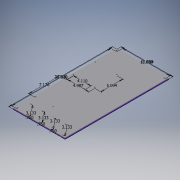
# Autodesk Inventor part: eboardbaseplate
Saved by Autodesk Inventor 2016 (Build 200138000, 138)
## iProperties
Created: 2016-01-21
Part Number: eboardbaseplate
Material: Generic
Document SubType Name: Modeling
Designer: Administrator
Density: 1 g/cm^3
Appearance: Default
Author: Administrator
Autodesk Inventor part; units mm, degrees
ref_plane "YZ Plane" through (0, 0, 0) normal (1, 0, 0) x (0, 1, 0)
ref_plane "XZ Plane" through (0, 0, 0) normal (0, 1, 0) x (-1, 0, 0)
ref_plane "XY Plane" through (0, 0, 0) normal (0, 0, 1) x (1, 0, 0)
sketch "Sketch1" plane through (0, 0, 0) normal (0, 1, 0) x (-1, 0, 0)
  line L0 (-139.7, 292.1) -> (139.7, 292.1)
  line L1 (139.7, 292.1) -> (139.7, -292.1)
  line L2 (139.7, -292.1) -> (-139.7, -292.1)
  line L3 (-139.7, -292.1) -> (-139.7, -89.789)
  line L4 (-139.7, 292.1) -> (139.7, -292.1) construction
  line L5 (139.7, 292.1) -> (-139.7, -292.1) construction
  line L6 (-152.4, 304.8) -> (152.4, 304.8)
  line L7 (152.4, 304.8) -> (152.4, -304.8)
  line L8 (152.4, -304.8) -> (-152.4, -304.8)
  line L9 (-152.4, -304.8) -> (-152.4, -89.789)
  line L10 (-152.4, 304.8) -> (152.4, -304.8) construction
  line L11 (152.4, 304.8) -> (-152.4, -304.8) construction
  line L12 (40.5945, 180.2806) -> (144.9885, 180.2806)
  line L13 (144.9885, 180.2806) -> (144.9885, -1.9898)
  line L14 (144.9885, -1.9898) -> (40.5945, -1.9898)
  line L15 (40.5945, -1.9898) -> (40.5945, 180.2806)
  line L16 (40.5945, 180.2806) -> (144.9885, -1.9898) construction
  line L17 (144.9885, 180.2806) -> (40.5945, -1.9898) construction
  line L18 (145.8849, -184.8763) -> (19.2151, -184.8763)
  line L19 (19.2151, -184.8763) -> (19.2151, -55.4887)
  line L20 (19.2151, -55.4887) -> (145.8849, -55.4887)
  line L21 (145.8849, -55.4887) -> (145.8849, -184.8763)
  line L22 (145.8849, -184.8763) -> (19.2151, -55.4887) construction
  line L23 (19.2151, -184.8763) -> (145.8849, -55.4887) construction
  line L24 (122.3815, 294.9298) -> (73.9219, 294.9298)
  line L25 (73.9219, 294.9298) -> (73.9219, 231.8081)
  line L26 (73.9219, 231.8081) -> (122.3815, 231.8081)
  line L27 (122.3815, 231.8081) -> (122.3815, 294.9298)
  line L28 (122.3815, 294.9298) -> (73.9219, 231.8081) construction
  line L29 (54.8719, 294.9298) -> (6.4122, 294.9298)
  line L30 (6.4122, 294.9298) -> (6.4122, 231.8081)
  line L31 (6.4122, 231.8081) -> (54.8719, 231.8081)
  line L32 (54.8719, 231.8081) -> (54.8719, 294.9298)
  line L33 (-12.6378, 294.9298) -> (-61.0974, 294.9298)
  line L34 (-61.0974, 294.9298) -> (-61.0974, 231.8081)
  line L35 (-61.0974, 231.8081) -> (-12.6378, 231.8081)
  line L36 (-12.6378, 231.8081) -> (-12.6378, 294.9298)
  line L37 (-80.1474, 294.9298) -> (-128.607, 294.9298)
  line L38 (-128.607, 294.9298) -> (-128.607, 231.8081)
  line L39 (-128.607, 231.8081) -> (-80.1474, 231.8081)
  line L40 (-80.1474, 231.8081) -> (-80.1474, 294.9298)
  line L41 (73.9219, 294.9298) -> (122.3815, 231.8081)
  line L42 (6.4122, 294.9298) -> (54.8719, 231.8081)
  line L43 (-61.0974, 294.9298) -> (-12.6378, 231.8081)
  line L44 (-128.607, 294.9298) -> (-80.1474, 231.8081)
  line L45 (139.7, -18.3929) -> (25.4, -18.3929)
  line L46 (25.4, -18.3929) -> (25.4, -208.8929)
  line L47 (25.4, -208.8929) -> (139.7, -208.8929)
  line L48 (139.7, -208.8929) -> (139.7, -18.3929)
  line L49 (-76.2, -89.789) -> (-152.4, -89.789)
  line L50 (-76.2, 89.789) -> (-76.2, -89.789)
  line L51 (-152.4, 89.789) -> (-76.2, 89.789)
  line L52 (-139.7, 89.789) -> (-139.7, 292.1)
  line L53 (-152.4, 89.789) -> (-152.4, 304.8)
  point P0 (0, 0)
  point P1 (0, 0)
  point P2 (0, 0)
  point P3 (92.7915, 89.1454)
  point P4 (92.7915, 89.1454)
  point P5 (82.55, -120.1825)
  point P6 (82.55, -120.1825)
  point P7 (98.1517, 263.3689)
  point P8 (82.55, -120.1825)
  point P9 (-152.4, 0)
  dimension "d71" = 279.4
  dimension "d72" = 584.2
  dimension "d73" = 304.8
  dimension "d74" = 609.6
  dimension "d84" = 104.394
  dimension "d85" = 182.2704
  dimension "d86" = 126.6698
  dimension "d87" = 129.3876
  dimension "d102" = 19.05
  dimension "d103" = 19.05
  dimension "d104" = 19.05
  dimension "d112" = 79.5782
  dimension "d113" = 79.5782
  dimension "d114" = 79.5782
  dimension "d115" = 79.5782
  dimension "d116" = 114.3
  dimension "d117" = 190.5
  dimension "d127" = 179.578
  dimension "d128" = 76.2
  dimension "d129" = 76.2
  dimension "d130" = 52.486
  dimension "d131" = 503.8227
  dimension "d132" = 440.701
  dimension "d133" = 503.8227
  dimension "d134" = 298.6819
  dimension "d135" = 30.0185
  dimension "d136" = 472.2618
  dimension "d137" = 12.7
  constraints: 108 end point, 24 coincident, 23 parallel, 14 midpoint, 11 horizontal, 9 perpendicular, 6 point on line, 3 other
  measures "d71" distance of L1.end L2.end
  measures "d72" distance of L0.end L1.end
  measures "d73" distance of L7.end L8.end
  measures "d74" distance of L6.end L7.end
  measures "d84" distance of L13.end L14.end
  measures "d85" distance of L12.end L13.end
  measures "d86" distance of L19.end L20.end
  measures "d87" distance of L18.end L19.end
  measures "d102" distance of L29.start L24.end
  measures "d103" distance of L33.start L29.end
  measures "d104" distance of L37.start L33.end
  measures "d112" distance of L41.start L41.end
  measures "d113" distance of L31.end L29.end
  measures "d114" distance of L35.end L33.end
  measures "d115" distance of L39.end L37.end
  measures "d116" distance of L47.end L46.end
  measures "d117" distance of L46.end L45.end
  measures "d127" distance of L50.start L49.start
  measures "d128" distance of L51.start L50.start
  measures "d129" distance of L49.start L9.end
  measures "d130" angle of L47 L28
  measures "d131" distance between parallel lines of L47 L24
  measures "d132" distance between parallel lines of L47 L31
  measures "d133" distance between parallel lines of L47 L33
  measures "d134" distance between parallel lines of L47 L51
  measures "d135" distance between parallel lines of L27 L7
  measures "d136" distance from line of point (98.152, 263.369) L47
  measures "d137" distance between parallel lines of L53 L52
extrude "Extrusion6" add sketch "Sketch1" along normal blind 6.35 contours L52 L51 L53 L6 L7 L8 L9 L49 L3 L2 L1 L18 L21 L20 L14 L13 L12 L0 L27 L24 L25 L32 L29 L30 L36 L33 L34 L40 L37 L38 | L0 L38 L39 L40 L34 L35 L36 L30 L31 L32 L25 L26 L27 L1 L12 L15 L14 L45 L46 L20 L19 L18 L47 L2 L3 L49 L50 L51 L52 | L38 L44 L0 | L0 L44 L39 L38 | L44 L37 L40 L0 | L0 L40 L44 | L34 L43 L0 | L0 L43 L35 L34 | L43 L33 L36 L0 | L0 L36 L43 | L30 L42 L0 | L0 L42 L31 L30 | L42 L29 L32 L0 | L0 L32 L42 | L1 L20 L21 L18 | L18 L19 L20 L46 | L25 L41 L0 | L0 L41 L26 L25 | L41 L24 L27 L0 | L0 L27 L41 | L14 L15 L12 L1 | L1 L12 L13 L14
hole "Hole6" at (139.7, 0, 292.1) at (-139.7, 0, 292.1) at (-139.7, 0, -292.1) at (139.7, 0, -292.1) at (-19.2151, 0, -55.4887) at (-19.2151, 0, -184.8763) at (-145.8849, 0, -184.8763) at (-145.8849, 0, -55.4887) at (-144.9885, 0, 180.2806) at (-40.5945, 0, 180.2806) at (-40.5945, 0, -1.9898) at (-144.9885, 0, -1.9898) direction (0, 1, 0) diameter 6.35 end through all
hole "Hole7" at (-122.3815, 0, 231.8081) at (-73.9219, 0, 294.9298) at (-54.8719, 0, 231.8081) at (-6.4122, 0, 294.9298) at (12.6378, 0, 231.8081) at (61.0974, 0, 294.9298) at (80.1474, 0, 231.8081) at (128.607, 0, 294.9298) direction (0, 1, 0) diameter 3.81 end through all
hole "Hole8" at (-139.7, 0, -18.3929) at (-25.4, 0, -18.3929) at (-25.4, 0, -208.8929) at (-139.7, 0, -208.8929) direction (0, 1, 0) diameter 6.35 end through all
body "Solid6"
